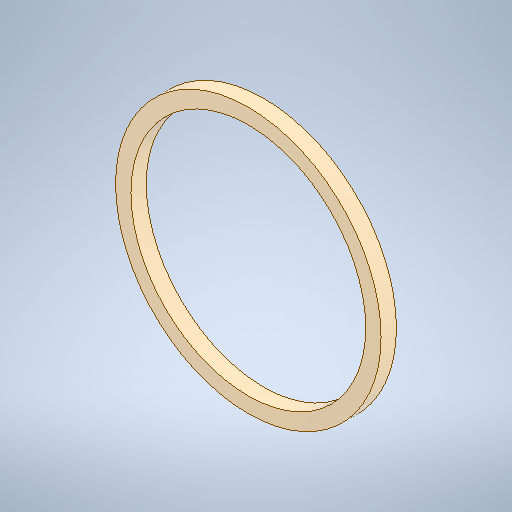
# Autodesk Inventor part: pierśnień
Saved by Autodesk Inventor 2025 (Build 290162000, 162)
## iProperties
Created: 2025-03-23
Part Number: pierśnień
Material: Polietylen o dużej gęstości
Document SubType Name: Modeling
Designer: barte
Density: 0.952 g/cm^3
Appearance: Gładki — w kolorze złamanej bieli
Author: barte
Autodesk Inventor part; units mm, degrees
ref_plane "YZ Plane" through (0, 0, 0) normal (1, 0, 0) x (0, 1, 0)
ref_plane "XZ Plane" through (0, 0, 0) normal (0, 1, 0) x (-1, 0, 0)
ref_plane "XY Plane" through (0, 0, 0) normal (0, 0, 1) x (1, 0, 0)
sketch "Szkic1" plane through (0, 0, 0) normal (0, 1, 0) x (-1, 0, 0)
  line L0 (34.6, 4.669) -> (30.6, 4.669)
  line L1 (30.6, 4.669) -> (30.6, 0.669)
  line L2 (30.6, 0.669) -> (34.6, 0.669)
  line L3 (34.6, 0.669) -> (34.6, 4.669)
  line L4 (0, 0) -> (0, 4)
  dimension "d1" = 4
  dimension "d2" = 4
  dimension "d3" = 4
  dimension "d4" = 4
  constraints: 10 end point, 1 perpendicular, 1 vertical
  measures "d1" distance of L0.start L0.end
  measures "d2" distance of L0.end L1.end
  measures "d3" distance of L1.end L2.end
  measures "d4" distance of L4.start L4.end
revolve "Obrót1" add sketch "Szkic1" angle 360 about axis through (0, 0, 0) along (0, 0, 1)
